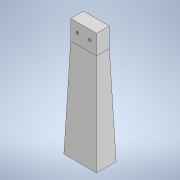
# Autodesk Inventor part: 限位開關架
Saved by Autodesk Inventor 2021 (Build 250183000, 183)
## iProperties
Created: 2023-02-07
Part Number: 限位開關架
Material: 一般
Document SubType Name: Modeling
Designer: brian
Density: 1 g/cm^3
Appearance: 預設
Author: brian
Autodesk Inventor part; units mm, degrees
ref_plane "YZ Plane" through (0, 0, 0) normal (1, 0, 0) x (0, 1, 0)
ref_plane "XZ Plane" through (0, 0, 0) normal (0, 1, 0) x (-1, 0, 0)
ref_plane "XY Plane" through (0, 0, 0) normal (0, 0, 1) x (1, 0, 0)
sketch "草圖1" plane through (0, 0, 0) normal (0, 1, 0) x (-1, 0, 0)
  line L0 (12.5, 7.5) -> (-12.5, 7.5)
  line L1 (-12.5, 7.5) -> (-12.5, -7.5)
  line L2 (-12.5, -7.5) -> (12.5, -7.5)
  line L3 (12.5, -7.5) -> (12.5, 7.5)
  line L4 (12.5, 7.5) -> (-12.5, -7.5) construction
  line L5 (-12.5, 7.5) -> (12.5, -7.5) construction
  point P0 (0, 0)
  dimension "d0" = 25
  dimension "d1" = 15
  constraints: 12 end point, 2 midpoint, 2 parallel, 1 horizontal, 1 perpendicular
  measures "d0" distance of L2.end L1.end
  measures "d1" distance of L1.end L0.end
extrude "擠出1" add sketch "草圖1" along normal blind 75 draft -2
sketch "草圖2" plane through (0, 75, 0) normal (0, 1, 0) x (1, 0, 0)
  line L0 (9.8809, -4.8809) -> (-9.8809, -4.8809) projected
  line L1 (9.8809, 4.8809) -> (9.8809, -4.8809) projected
  line L2 (-9.8809, 4.8809) -> (9.8809, 4.8809) projected
  line L3 (-9.8809, -4.8809) -> (-9.8809, 4.8809) projected
  point P0 (0, 0)
extrude "擠出2" add sketch "草圖2" along normal blind 15
sketch "草圖3" plane through (9.8809, 75, -4.8809) normal (0, 0, -1) x (-1, 0, 0)
  line L0 (19.7619, 0) -> (0, 0) projected
  line L1 (19.7619, 0) -> (19.7619, 15) projected
  line L2 (0, 15) -> (19.7619, 15) projected
  line L3 (0, 0) -> (0, 15) projected
  line L4 (0, 15) -> (19.7619, 15) projected
  line L5 (5.1309, 15) -> (14.6309, 15)
  line L6 (14.6309, 15) -> (14.6309, 8)
  line L7 (14.6309, 8) -> (5.1309, 8)
  line L8 (5.1309, 8) -> (5.1309, 15)
  point P0 (9.8809, -75)
  point P1 (9.8809, 8)
  point P2 (9.8809, 15)
  dimension "d6" = 9.5
  dimension "d7" = 7
  constraints: 8 end point, 2 coincident, 2 midpoint, 2 parallel, 1 horizontal, 1 perpendicular, 1 point on line, 1 vertical alignment
  measures "d6" distance of L6.end L7.end
  measures "d7" distance of L5.end L6.end
hole "孔1" at (4.75, 83, -4.8809) at (-4.75, 83, -4.8809) direction (0, 0, 1) diameter 2 end through all counterbore diameter 3.25 counterbore depth 5.8
sketch "草圖4" plane through (0, 0, 0) normal (0, -1, 0) x (1, 0, 0)
  point P0 (0, 0)
  point P1 (5, 0)
  point P2 (-5, 0)
  dimension "d15" = 10
  dimension "d16" = 5
  constraints: 2 horizontal alignment
  measures "d15" distance of point (-5, 0) point (5, 0)
  measures "d16" distance of point (0, 0) point (5, 0)
hole "孔2" at (5, 0, 0) at (-5, 0, 0) direction (0, 1, 0) diameter 2.7 depth 20 counterbore diameter 4.1 counterbore depth 6
equation "\"d16\" = 0.5 * d15"
